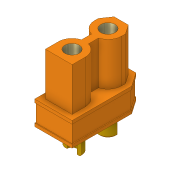
# Autodesk Inventor part: stecker2
Saved by Autodesk Inventor 2017 (Build 210142000, 142)
## iProperties
Part Number: stecker2
Material: Generisch
Document SubType Name: Modeling
Designer: ExCISS
Density: 1 g/cm^3
Appearance: Vorgabe
Author: ExCISS
Autodesk Inventor part; units mm, degrees
ref_plane "YZ Plane" through (0, 0, 0) normal (1, 0, 0) x (0, 1, 0)
ref_plane "XZ Plane" through (0, 0, 0) normal (0, 1, 0) x (-1, 0, 0)
ref_plane "XY Plane" through (0, 0, 0) normal (0, 0, 1) x (1, 0, 0)
sketch "Skizze1" plane through (0, 0, 0) normal (0, 0, 1) x (1, 0, 0)
  line L0 (-2.6, -5.1) -> (2.6, -5.1)
  line L1 (2.6, -5.1) -> (2.6, 3.2)
  line L2 (-2.6, -5.1) -> (-2.6, 3.2)
  line L3 (-1.3, 5.1) -> (1.3, 5.1)
  line L4 (0, -5.1) -> (0, 5.1) construction
  line L5 (-2.6, 3.2) -> (-1.3, 5.1)
  line L6 (1.3, 5.1) -> (2.6, 3.2)
  point P0 (0, 0)
  point P1 (0, 0)
  dimension "d0" = 5.2
  dimension "d1" = 8.3
  dimension "d2" = 2.6
  dimension "d3" = 10.2
  constraints: 14 end point, 3 midpoint, 2 horizontal, 2 vertical, 1 coincident, 1 parallel, 1 perpendicular
  measures "d0" distance of L0.start L0.end
  measures "d1" distance of L0.end L1.end
  measures "d2" distance of L3.start L3.end
  measures "d3" distance of L4.end L4.start
extrude "Extrusion1" add sketch "Skizze1" along normal blind 3.33
sketch "Skizze3" plane through (0, 0, 3.33) normal (0, 0, 1) x (1, 0, 0)
  line L0 (0, -0.674) -> (0, 0.674) construction
  line L1 (0, 0) -> (0, 4.35) construction
  line L2 (-0.989, 4.35) -> (0.989, 4.35)
  line L3 (0.989, 4.35) -> (1.8672, 3.0665)
  line L4 (-0.989, 4.35) -> (-1.8885, 3.0353)
  line L5 (-1.3, 5.1) -> (-2.6, 3.2) projected
  line L6 (2.6, 3.2) -> (1.3, 5.1) projected
  circle A0 centre (0, 2.5) radius 0.5 construction
  circle A1 centre (0, 2.5) radius 0.5 construction
  line L7 (-1.8885, 3.0353) -> (-1.8885, 2.5219)
  line L8 (1.8672, 3.0665) -> (1.8672, 2.5531)
  arc A2 (-1.8885, 2.5219) -> (1.8672, 2.5531) centre (-0.0105, 2.5219) ccw
  dimension "d11" = 1.348
  dimension "d12" = 4.35
  dimension "d13" = 1.978
  constraints: 14 end point, 4 vertical, 3 parallel, 2 midpoint, 2 point on circle, 1 centre point, 1 coincident, 1 horizontal, 1 tangent
  measures "d11" distance of L0.start L0.end
  measures "d12" distance of L1.end L1.start
  measures "d13" distance of L2.start L2.end
extrude "Extrusion3" add sketch "Skizze3" along normal blind 6
sketch "Skizze4" plane through (0, 0, 3.33) normal (0, 0, 1) x (1, 0, 0)
  line L0 (-2.6, 3.2) -> (-2.6, -5.1) construction
  line L1 (-2.6, -4.6629) -> (-2.6, -0.9339) construction
  line L2 (-1.8645, -4.35) -> (1.8645, -4.35)
  arc A0 (-1.8885, 2.5219) -> (1.8672, 2.5531) centre (-0.0105, 2.5219) ccw projected
  line L3 (-1.8645, -4.35) -> (-1.8645, -2.5085)
  line L4 (1.8645, -4.35) -> (1.8645, -2.5085)
  arc A1 (1.8645, -2.5085) -> (-1.8645, -2.5085) centre (0, -2.5085) ccw
  line L5 (-0.4867, 0.8046) -> (0.4867, 0.8046)
  line L6 (0.4867, 0.8046) -> (0.4867, -0.8046)
  line L7 (0.4867, -0.8046) -> (-0.4867, -0.8046)
  line L8 (-0.4867, -0.8046) -> (-0.4867, 0.8046)
  line L9 (-0.4867, 0.8046) -> (0.4867, -0.8046) construction
  point P0 (0, 0)
  point P1 (0, 0)
  dimension "d18" = 3.729
  constraints: 18 end point, 3 parallel, 2 horizontal, 2 point on circle, 2 point on line, 2 tangent, 2 vertical, 1 centre point, 1 coincident, 1 midpoint, 1 perpendicular
  measures "d18" distance of L2.start L2.end
extrude "Extrusion4" add sketch "Skizze4" along normal blind 6
sketch "Skizze5" plane through (0, 0, 9.33) normal (0, 0, 1) x (1, 0, 0)
  line L0 (0, -2.5) -> (0, 2.5) construction
  circle A0 centre (0, 2.5) radius 1
  circle A1 centre (0, -2.5) radius 1
  point P0 (0, 0)
  point P1 (0, 0)
  point P2 (0, 0)
  dimension "d22" = 5
  dimension "d23" = 2
  dimension "d24" = 2
  constraints: 3 coincident, 2 centre point, 2 end point, 1 midpoint, 1 vertical
  measures "d22" distance of L0.start L0.end
  measures "d23" diameter of A0
  measures "d24" diameter of A1
extrude "Extrusion5" cut sketch "Skizze5" against normal blind 6
sketch "Skizze6" plane through (2.6, -5.1, 0) normal (1, 0, 0) x (0, 0, -1)
  line L0 (-3.33, 4.3914) -> (-9.33, 4.3914) construction
  line L1 (-3.33, 4.3914) -> (-2.88, 4.3914) construction
  line L2 (0, 5.1) -> (-0.45, 5.1) construction
  line L3 (0, 0) -> (-3.33, 0) projected
  line L4 (0, 8.3) -> (-3.33, 8.3) projected
  line L5 (-2.88, 0) -> (-0.45, 0)
  line L6 (-0.45, 0) -> (-0.45, 8.3)
  line L7 (-0.45, 8.3) -> (-2.88, 8.3)
  line L8 (-2.88, 8.3) -> (-2.88, 0)
  dimension "d31" = 0.45
  dimension "d32" = 0.45
  constraints: 12 end point, 3 horizontal, 2 parallel, 2 point on line, 1 perpendicular
  measures "d31" distance of L0.start L1.end
  measures "d32" distance of L2.start L2.end
extrude "Extrusion6" cut sketch "Skizze6" against normal blind 0.1
sketch "Skizze7" plane through (1.3, 5.1, 3.33) normal (0.8253, 0.5647, 0) x (0, 0, -1)
  line L0 (0.45, -2.3022) -> (0, -2.3022) projected
  line L1 (3.33, 0) -> (0, 0) projected
  line L2 (0.45, -2.3022) -> (2.8887, -2.3022)
  line L3 (2.8887, -2.3022) -> (2.8887, 0)
  line L4 (2.8887, 0) -> (0.45, 0)
  line L5 (0.45, 0) -> (0.45, -2.3022)
  point P0 (3.33, -3.475)
  constraints: 8 end point, 2 parallel, 1 horizontal, 1 perpendicular, 1 point on line
extrude "Extrusion7" cut sketch "Skizze7" against normal blind 0.1
sketch "Skizze8" plane through (-1.3, 5.1, 0) normal (0, 1, 0) x (1, 0, 0)
  line L0 (2.6, -2.88) -> (2.6, -3.33) projected
  line L1 (0, 0) -> (0, -3.33) projected
  line L2 (2.6, -2.88) -> (0, -2.88)
  line L3 (0, -2.88) -> (0, -0.4356)
  line L4 (0, -0.4356) -> (2.6, -0.4356)
  line L5 (2.6, -0.4356) -> (2.6, -2.88)
  point P0 (1.3, 0)
  constraints: 8 end point, 2 parallel, 1 horizontal, 1 perpendicular, 1 point on line
extrude "Extrusion8" cut sketch "Skizze8" against normal blind 0.1
sketch "Skizze9" plane through (-2.6, 3.2, 0) normal (-0.8253, 0.5647, 0) x (0, 0, 1)
  line L0 (2.88, 3.7704) -> (2.88, 2.3022) projected
  line L1 (0, 0) -> (3.33, 0) projected
  line L2 (2.88, 2.3022) -> (0.436, 2.3022)
  line L3 (0.436, 2.3022) -> (0.436, 0)
  line L4 (0.436, 0) -> (2.88, 0)
  line L5 (2.88, 0) -> (2.88, 2.3022)
  point P0 (0, -1.1728)
  dimension "d39" = 2.444
  constraints: 8 end point, 2 parallel, 1 horizontal, 1 perpendicular, 1 point on line
  measures "d39" distance of L4.end L3.end
extrude "Extrusion9" cut sketch "Skizze9" against normal blind 0.1
sketch "Skizze10" plane through (-2.6, -5.1, 0) normal (-1, 0, 0) x (0, 0, 1)
  line L0 (0.4366, 8.3229) -> (2.8806, 8.3229)
  line L1 (2.8806, 8.3229) -> (2.8806, 0)
  line L2 (2.8806, 0) -> (0.4366, 0)
  line L3 (0.4366, 0) -> (0.4366, 8.3229)
  point P0 (0, 5.1)
  dimension "d42" = 2.444
  constraints: 8 end point, 2 parallel, 1 horizontal, 1 perpendicular
  measures "d42" distance of L1.end L2.end
extrude "Extrusion10" cut sketch "Skizze10" against normal blind 0.1
sketch "Skizze11" plane through (-2.6, -5.1, 0) normal (0, -1, 0) x (1, 0, 0)
  line L0 (1.3, 2.88) -> (0.0157, 2.88) projected
  line L1 (3.8473, 0.4413) -> (5.1175, 0.4413) projected
  line L2 (0.0989, 2.88) -> (5.1175, 2.88)
  line L3 (5.1175, 2.88) -> (5.1175, 0.4413)
  line L4 (5.1175, 0.4413) -> (0.0989, 0.4413)
  line L5 (0.0989, 0.4413) -> (0.0989, 2.88)
  point P0 (2.6, 0)
  constraints: 8 end point, 2 parallel, 1 horizontal, 1 perpendicular, 1 point on line
extrude "Extrusion11" cut sketch "Skizze11" against normal blind 0.1
sketch "Skizze12" plane through (0, 0, 0) normal (0, 0, -1) x (-1, 0, 0)
  circle A0 centre (0, -2.5) radius 1 construction
  circle A1 centre (0, -2.5) radius 1 construction
  circle A2 centre (0, 2.5) radius 1 construction
  circle A3 centre (0, 2.5) radius 1 construction
  circle A4 centre (0, -2.5) radius 1.3
  circle A5 centre (0, 2.5) radius 1.3
  point P0 (0, 0)
  dimension "d47" = 2.6
  constraints: 2 centre point, 2 coincident, 1 equal radius
  measures "d47" diameter of A4
extrude "Extrusion12" add sketch "Skizze12" along normal blind 3
chamfer "Fase1" distance 0.2 angle 45 2 edges at (1.3, -2.5, -3) (1.3, 2.5, -3)
sketch "Skizze13" plane through (0, -2.5, -3) normal (0, 0, -1) x (-1, 0, 0)
  circle A0 centre (0, 0) radius 1.1 projected
  circle A1 centre (0, 5) radius 1.1 projected
  point P0 (0, 2.5)
hole "Bohrung1" at (0, 2.5, -3) at (0, -2.5, -3) direction (0, 0, 1) diameter 1.4 depth 4.5 tip angle 118
sketch "Skizze14" plane through (0, -2.5, -3) normal (0, 0, -1) x (-1, 0, 0)
  circle A0 centre (0, 0) radius 1.3 construction
  circle A1 centre (0, 5) radius 1.3 construction
  line L0 (2.6, -2.6) -> (-2.6, -2.6) construction
  line L1 (2.6, 5.7) -> (2.6, -2.6) construction
  line L2 (1.3, 7.6) -> (2.6, 5.7) construction
  line L3 (-1.3, 7.6) -> (1.3, 7.6) construction
  line L4 (-2.6, 5.7) -> (-1.3, 7.6) construction
  line L5 (-2.6, -2.6) -> (-2.6, 5.7) construction
  line L6 (-1.3, 0) -> (1.3, 0)
  line L7 (-1.3, 5) -> (1.3, 5)
  circle A2 centre (0, 0) radius 1.3 projected
  arc A3 (-1.3, 0) -> (1.3, 0) centre (0, 0) ccw
  circle A4 centre (0, 5) radius 0.7 projected
  arc A5 (1.3, 5) -> (-1.3, 5) centre (0, 5) ccw
  point P0 (0, 2.5)
  constraints: 4 coincident, 4 end point, 4 point on circle, 2 centre point, 2 horizontal, 2 horizontal alignment, 2 midpoint, 2 other
extrude "Extrusion13" cut sketch "Skizze14" against normal blind 2.5 contours L6 A2 | A4 L7 A5 | L7 A4 picked at (-0.4207, -0.1037) picked at (0.2266, 5.0558)
